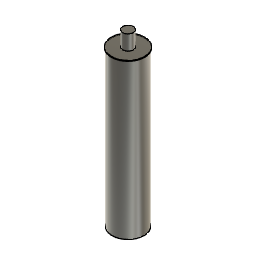
stick v4 (Autodesk Fusion 360 design; units mm, degrees)
Autodesk Fusion 360 part; units mm, degrees
sketch "Sketch1" plane through (0, 0, 0) normal (0, 0, 1) x (1, 0, 0)
  line L0 (0, 0) -> (0, 2.5)
  line L1 (0, 0) -> (2.1651, -1.25)
  arc A0 (2.1651, -1.25) -> (0, 2.5) centre (0, 0) ccw
  dimension "d9" = 120
  dimension "d10" = 2.5
  constraint vertical L0
  constraint coincident L0.start L1.start
  constraint vertical L0.start L0.end
  measures "d9" angle of L0 L1
  measures "d10" distance of L1 A0
extrude "Extrude1" add sketch "Sketch1" along normal blind 5 and the other way blind 2 makes body 1
sketch "Sketch2" plane through (0, 0, 5) normal (0, 0, 1) x (-1, 0, 0)
  line L0 (0, 0) -> (-2.1651, 1.25)
  arc A0 (-2.1651, 1.25) -> (0, -2.5) centre (0, 0) ccw
  line L1 (0, -2.5) -> (0, 0)
  line L2 (0, 0) -> (0, -7.5)
  line L3 (0, 0) -> (-6.4952, 3.75)
  arc A1 (-6.4952, 3.75) -> (0, -7.5) centre (0, 0) ccw
  dimension "d11" = 7.5
  constraint coincident L1 L0.start
  constraint coincident L0.start A0.centre
  constraint coincident A0.end L2
  constraint coincident L0.end L3
  measures "d11" radius of A1
extrude "Extrude2" add sketch "Sketch2" along normal blind 75 bodies 1
move_body "Move1" bodies 1 to x (-1, 0, 0) y (0, 1, 0) z (0, 0, -1) at (0, 0, 0)
move_body "Move2" bodies 1 to x (1, 0, 0) y (0, 1, 0) z (0, 0, 1) at (0, 0, 80)
sketch "Sketch3" plane through (0, 0, 0) normal (0.5, -0.866025, 0) x (0.866025, 0.5, 0)
  line L0 (-2.5, 82) -> (-2.5, 75)
  line L1 (-2.5, 75) -> (-7.5, 75)
  line L2 (-7.5, 75) -> (-7.5, 0)
  line L3 (-7.5, 0) -> (0, 0)
  line L4 (0, 0) -> (0, 82)
  line L5 (0, 82) -> (-2.5, 82)
  line L6 (-7.5, 75) -> (-7.85, 75)
  line L7 (-7.85, 75) -> (-7.85, 74.65)
  line L8 (-7.85, 74.65) -> (-7.5, 74.65)
  line L9 (-7.5, 74.65) -> (-7.5, 75)
  dimension "d13" = 0.35
  constraint horizontal L6
  constraint vertical L7
  constraint horizontal L8
  constraint vertical L9
  constraint coincident L1.end L2.start
  constraint equal L6 L7
  measures "d13" distance of L6.end L7.end
sweep "Sweep1" add profiles "Sketch3" along 1 edges at (-6.4952, 3.75, 75) section 1 contours L2 L6 L7 L8 L9 on bodies 1 bodies 1
extrude "Extrude3" cut 1 faces at (-0.3726, 4.9721, 0) along direction (0, 0, 1) blind 2 on bodies 1 bodies 1
move_body "Move3" bodies 1 to x (1, 0, 0) y (0, 1, 0) z (0, 0, 1) at (0, 0, -2)
pattern_circular "C-Pattern1" count 3 over 360 about axis through (0, 0, 0) along (0, 0, 1) of bodies 1 makes body 2 at (-6.3002, -4.0691, 24.2167) makes body 3 at (6.674, -3.4216, 24.2167)
combine "Combine1" operation add target body 1 tool bodies 3 2
